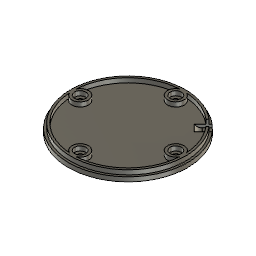
Wifi_top_cover (Autodesk Fusion 360 design; units mm, degrees)
part number: 2026-05-21-09-43-14-642
Autodesk Fusion 360 part; units mm, degrees
sketch "Sketch1" plane through (0, 0, 0) normal (0, 0, 1) x (1, 0, 0)
  circle A0 centre (0, 0) radius 40
  dimension "d1" = 80
  constraint coincident A0.centre origin
  measures "d1" diameter of A0
extrude "Extrude1" add sketch "Sketch1" along normal blind 3
sketch "Sketch2" plane through (0, 0, 3) normal (0, 0, 1) x (-1, 0, 0)
  circle A0 centre (0, 0) radius 40
  circle A1 centre (0, 0) radius 38.5
  circle A2 centre (0, 32) radius 3.75
  circle A3 centre (0, 32) radius 5.5
  circle A4 centre (0, 0) radius 37
  dimension "d4" = 77
  dimension "d5" = 7.5
  dimension "d6" = 11
  dimension "d7" = 32
  dimension "d8" = 74
  constraint coincident A0.centre A1.centre
  constraint concentric A2 A3
  measures "d4" diameter of A1
  measures "d5" diameter of A2
  measures "d6" diameter of A3
  measures "d7" distance of A0.centre A2.centre
  measures "d8" diameter of A4
extrude "Extrude2" add sketch "Sketch2" along normal blind 3 contours A1 | A3 A4 | A3 A4 picked at (-1.5513, 36.4665) picked at (0.1215, 37.1566)
pattern_circular "C-Pattern1" count 4 over 360 about axis through (0, 0, 1.75) along (0, 0, 1) of "Extrude2"
sketch "Sketch3" plane through (0, 0, 0) normal (0, 0, -1) x (1, 0, 0)
  circle A0 centre (0, 0) radius 40
  circle A1 centre (0, -32) radius 3
  dimension "d13" = 6
  dimension "d14" = 32
  measures "d13" diameter of A1
  measures "d14" distance of A0.centre A1.centre
extrude "Extrude3" cut sketch "Sketch3" against normal through all draft -25 contours A1
pattern_circular "C-Pattern2" count 4 over 360 about axis through (0, 0, 0) along (0, 0, 1) of "Extrude3"
ref_plane "WorkPlane1" through (0, 0, 0) normal (-0.707107, 0.707107, 0) x (0, 0, 1)
sketch "Sketch4" plane through (0, 0, 0) normal (-0.707107, 0.707107, 0) x (0, 0, 1)
  line L0 (6, -27.2236) -> (6, 38.5)
  line L1 (6, -38.5) -> (6, -27.2236)
  line L2 (3, -40) -> (3, -38.5)
  line L3 (3, 38.5) -> (3, 40)
  line L4 (0, -40) -> (0, 40)
  line L5 (3, -38.5) -> (6, -38.5)
  line L6 (3, 38.5) -> (6, 38.5)
  line L7 (0, -40) -> (3, -40)
  line L8 (0, 40) -> (3, 40)
  line L9 (3, 40) -> (6, 40)
  line L10 (6, 40) -> (6, 30.653)
  line L11 (3, 40) -> (1, 40)
  line L12 (1, 40) -> (1, 35.115)
  arc A0 (1, 35.115) -> (6, 30.653) centre (5.4909, 35.115) ccw
  dimension "d18" = 3
  dimension "d19" = 9.347
  dimension "d20" = 2
  dimension "d21" = 4.885
  constraint coincident L3.end L8.end
  constraint perpendicular L3 L9
  constraint perpendicular L9 L10
  constraint perpendicular L3 L11
  constraint perpendicular L11 L12
  constraint tangent L12 A0
  measures "d18" distance of L3.end L9.end
  measures "d19" distance of L9.end L10.end
  measures "d20" distance of L3.end L11.end
  measures "d21" distance of L11.end L12.end
extrude "Extrude4" cut sketch "Sketch4" along normal mid plane 6 contours L0 L3 L6 L8 L10 L11 L12 A0 | L3 L6 L9 L10
